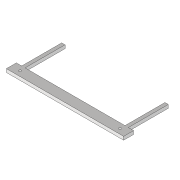
# Autodesk Inventor part: Gestell_Seite
Saved by Autodesk Inventor 2020 (Build 240168000, 168)
## iProperties
Created: 2020-03-18
Part Number: Gestell_Seite
Material: Generisch
Document SubType Name: Modeling
Designer: franz
Density: 1 g/cm^3
Appearance: Vorgabe
Author: franz
Autodesk Inventor part; units mm, degrees
ref_plane "YZ Plane" through (0, 0, 0) normal (1, 0, 0) x (0, 1, 0)
ref_plane "XZ Plane" through (0, 0, 0) normal (0, 1, 0) x (-1, 0, 0)
ref_plane "XY Plane" through (0, 0, 0) normal (0, 0, 1) x (1, 0, 0)
sketch "Skizze1" plane through (0, 0, 0) normal (0, 1, 0) x (-1, 0, 0)
  line L0 (800, 0) -> (800, -600)
  line L1 (800, -600) -> (750, -600)
  line L2 (750, -600) -> (750, 0)
  line L3 (750, 0) -> (-750, 0)
  line L4 (-750, 0) -> (-750, -600)
  line L5 (-750, -600) -> (-800, -600)
  line L6 (-800, -600) -> (-800, 0)
  line L7 (-800, 0) -> (-880, 0)
  line L8 (-880, 0) -> (-880, 150)
  line L9 (-880, 150) -> (880, 150)
  line L10 (880, 150) -> (880, 0)
  line L11 (880, 0) -> (800, 0)
  line L12 (0, -750) -> (0, 300) projected
  point P0 (0, 0)
  dimension "d0" = 50
  dimension "d1" = 600
  dimension "d2" = 150
  dimension "d3" = 1500
  dimension "d4" = 80
  constraints: 24 end point, 9 perpendicular, 5 point on line, 1 midpoint, 1 vertical, 3 other
  measures "d0" distance of L0.end L1.end
  measures "d1" distance between parallel lines of L3 L1
  measures "d2" distance of L9.end L10.end
  measures "d3" distance between parallel lines of L4 L2
  measures "d4" distance between parallel lines of L0 L10
extrude "Extrusion1" add sketch "Skizze1" along normal blind 50
sketch "Skizze2" plane through (0, 0, 0) normal (0, -1, 0) x (1, 0, 0)
  circle A0 centre (-750, 75) radius 42.5
  circle A1 centre (750, 75) radius 42.5
  line L0 (0, -750) -> (0, 300) projected
  line L1 (750, 0) -> (-750, 0) projected
  point P0 (0, 0)
  dimension "d7" = 85
  dimension "d8" = 85
  dimension "d9" = 1500
  dimension "d10" = 75
  constraints: 2 centre point, 1 symmetric about line
  measures "d7" diameter of A0
  measures "d8" diameter of A1
  measures "d9" distance of A0.centre A1.centre
  measures "d10" distance from line of A0.centre L1
extrude "Extrusion2" cut sketch "Skizze2" against normal blind 25
sketch "Skizze3" plane through (0, 50, 0) normal (0, 1, 0) x (1, 0, 0)
  circle A0 centre (750, -75) radius 42.5 projected
  circle A1 centre (-750, -75) radius 42.5 projected
  circle A2 centre (750, -75) radius 17.5
  circle A3 centre (-750, -75) radius 17.5
  point P0 (0, 0)
  dimension "d13" = 35
  dimension "d14" = 35
  constraints: 2 centre point, 2 coincident
  measures "d13" diameter of A2
  measures "d14" diameter of A3
extrude "Extrusion3" cut sketch "Skizze3" against normal through all contours A2 | A3
equation "\"d8\" = d7"
